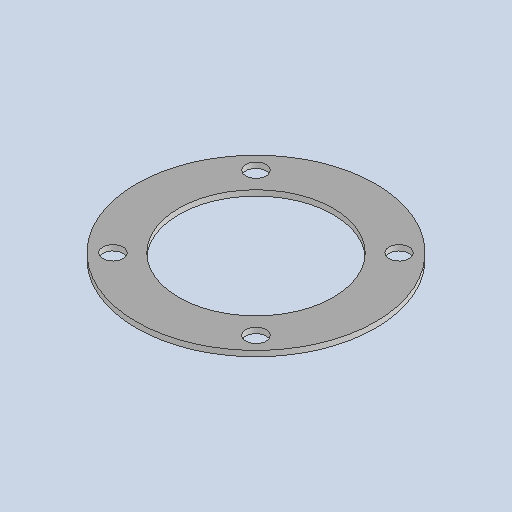
# Autodesk Inventor part: DSB 138 head loose flange
Saved by Autodesk Inventor 2025 (Build 290162010, 162A)
## iProperties
Created: 2024-12-09
Part Number: DSB 138 head loose flange
Material: Generic
Document SubType Name: Sheet Metal
Designer: user
Mass: 22.054 g
Surface Area: 171.342 cm^2
Volume: 22.054 cm^3
Density: 1 g/cm^3
Flat Pattern Width: 13 cm
Flat Pattern Length: 13 cm
Flat Pattern Area: 169 cm^2
Sheet Metal Rule: Default
Sheet Metal Width: 130,000 mm
Sheet Metal Length: 130,000 mm
Sheet Metal Area: 16900,000 mm^2
Appearance: Default
Octaeder_side: 55.919 mm
Octaeder_flange_lenth: 72.500 mm
Author: user
Autodesk Inventor part; units mm, degrees
ref_plane "YZ Plane" through (0, 0, 0) normal (1, 0, 0) x (0, 1, 0)
ref_plane "XZ Plane" through (0, 0, 0) normal (0, 1, 0) x (-1, 0, 0)
ref_plane "XY Plane" through (0, 0, 0) normal (0, 0, 1) x (1, 0, 0)
sketch "Sketch1" plane through (0, 0, 0) normal (0, 0, 1) x (1, 0, 0)
  circle A0 centre (0, 0) radius 42
  circle A1 centre (0, 0) radius 65
  line L0 (45.9619, -45.9619) -> (-45.9619, 45.9619) construction
  line L1 (-45.9619, -45.9619) -> (45.9619, 45.9619) construction
  point P0 (0, 42)
  dimension "d44" = 84
  dimension "d23" = 130
  measures "d23" diameter of A1
extrude "Plate1" add sketch "Sketch1" along normal blind 3
sketch "Sketch6" plane through (0, 0, 0) normal (0, 0, 1) x (1, 0, 0)
  line L0 (0, 0) -> (0, 55) construction
  circle A0 centre (0, 0) radius 55 construction
  line L1 (0, 0) -> (38.8909, 38.8909) construction
  circle A1 centre (38.8909, 38.8909) radius 5.5
  dimension "d42" = 72.5
  dimension "d32" = 11
  dimension "d33" = 110
  dimension "d34" = 45
  constraints: 4 end point, 2 centre point, 2 coincident, 2 point on circle, 1 vertical
  measures "d32" diameter of A1
  measures "d33" diameter of A0
  measures "d34" angle of L0 L1
extrude "Cut2" cut sketch "Sketch6" along normal blind 3
pattern_circular "Circular Pattern2" count 4 over 360 about axis through (0, 0, -10) along (0, 0, -1) of "Cut2"
equation "\"d35\" = Thickness"
equation "\"d2\" = Thickness"
equation "\"BendRadius\" = Thickness"
equation "\"BendReliefWidth\" = Thickness"
equation "\"BendReliefDepth\" = 0.5 * Thickness"
equation "\"CornerReliefSize\" = 4 * Thickness"
equation "\"MinimumRemnant\" = 2 * Thickness"
equation "\"TransitionRadius\" = BendRadius"
equation "\"JacobiRadiusSize\" = BendRadius"
equation "\"GapSize\" = Thickness"
equation "\"Octaeder_side\" = d41"
equation "\"Octaeder_flange_lenth\" = d42"
equation "\"Thickness\" = 3"
equation "\"d41\" = 55.918831"
body "Solid1"
